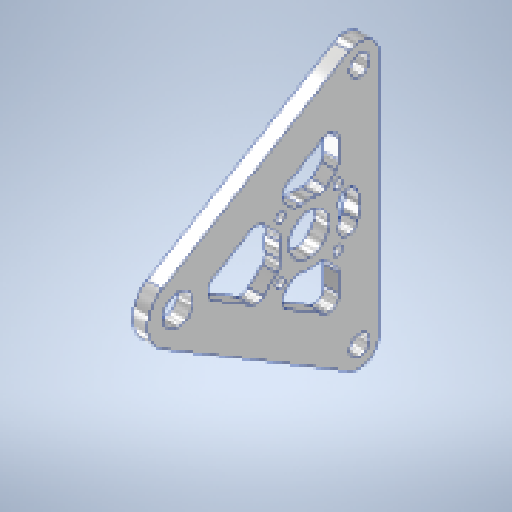
# Autodesk Inventor part: Frame (Motor Side)
Saved by Autodesk Inventor 2023.2 (Build 272271000, 271)
## iProperties
Created: 2022-05-22
Part Number: Frame (Motor Side)
Material: Aluminum 6061
Document SubType Name: Modeling
Designer: Nathan Cai
Density: 2.7 g/cm^3
Appearance: Aluminum - Flat
Mass: 51.1911 g
Surface Area: 97.1122 cm^2
Volume: 18.9597 cm^3
Author: Nathan Cai
Autodesk Inventor part; units mm, degrees
ref_plane "YZ Plane" through (0, 0, 0) normal (1, 0, 0) x (0, 1, 0)
ref_plane "XZ Plane" through (0, 0, 0) normal (0, 1, 0) x (-1, 0, 0)
ref_plane "XY Plane" through (0, 0, 0) normal (0, 0, 1) x (1, 0, 0)
sketch "Sketch1" plane through (0, 0, 0) normal (1, 0, 0) x (0, 1, 0)
  circle A0 centre (0, 0) radius 6.35
  circle A1 centre (0, 0) radius 22.225
  line L0 (0, 0) -> (0, 41.275) construction
  circle A2 centre (0, 41.275) radius 4.7625
  circle A3 centre (0, 41.275) radius 76.2 construction
  circle A4 centre (0, 41.275) radius 9.525
  line L1 (0, -15.875) -> (38.1, -15.875) construction
  circle A5 centre (38.1, -15.875) radius 3.175
  arc A6 (32.6593, -19.1494) -> (43.5407, -12.6006) centre (38.1, -15.875) ccw
  line L2 (8.161, 46.1865) -> (43.5407, -12.6006)
  line L3 (1.9103, 31.9435) -> (32.6593, -19.1494)
  circle A7 centre (-38.1, -15.875) radius 3.175
  arc A8 (-43.5407, -12.6006) -> (-32.6593, -19.1494) centre (-38.1, -15.875) ccw
  line L4 (-8.161, 46.1865) -> (-43.5407, -12.6006)
  line L5 (-1.9103, 31.9435) -> (-32.6593, -19.1494)
  line L6 (0, 0) -> (9.5, 0) construction
  line L7 (0, 0) -> (12.7, 0) construction
  line L8 (0, 0) -> (4.3437, -11.9341)
  line L9 (38.1, -15.875) -> (7.351, 35.2179) construction
  line L10 (-9, 9) -> (9, 9) construction
  arc A9 (3.287, 12.2673) -> (-3.287, 12.2673) centre (0, 0) ccw construction
  arc A10 (4.1088, 15.3341) -> (-4.1088, 15.3341) centre (0, 0) ccw
  arc A11 (2.4653, 9.2004) -> (-2.4653, 9.2004) centre (0, 0) ccw
  arc A12 (2.4653, 9.2004) -> (4.1088, 15.3341) centre (3.287, 12.2673) ccw
  arc A13 (-4.1088, 15.3341) -> (-2.4653, 9.2004) centre (-3.287, 12.2673) ccw
  line L11 (0, 0) -> (-3.287, 12.2673) construction
  line L12 (0, 0) -> (3.287, 12.2673) construction
  arc A14 (-9.2004, 2.4653) -> (-9.2004, -2.4653) centre (0, 0) ccw
  arc A15 (-9.2004, 2.4653) -> (-15.3341, 4.1088) centre (-12.2673, 3.287) ccw
  arc A16 (-15.3341, -4.1088) -> (-9.2004, -2.4653) centre (-12.2673, -3.287) ccw
  arc A17 (-12.2673, 3.287) -> (-12.2673, -3.287) centre (0, 0) ccw construction
  arc A18 (-15.3341, 4.1088) -> (-15.3341, -4.1088) centre (0, 0) ccw
  arc A19 (-2.4653, -9.2004) -> (2.4653, -9.2004) centre (0, 0) ccw
  arc A20 (-2.4653, -9.2004) -> (-4.1088, -15.3341) centre (-3.287, -12.2673) ccw
  arc A21 (4.1088, -15.3341) -> (2.4653, -9.2004) centre (3.287, -12.2673) ccw
  arc A22 (-3.287, -12.2673) -> (3.287, -12.2673) centre (0, 0) ccw construction
  arc A23 (-4.1088, -15.3341) -> (4.1088, -15.3341) centre (0, 0) ccw
  arc A24 (9.2004, -2.4653) -> (9.2004, 2.4653) centre (0, 0) ccw
  arc A25 (9.2004, -2.4653) -> (15.3341, -4.1088) centre (12.2673, -3.287) ccw
  arc A26 (15.3341, 4.1088) -> (9.2004, 2.4653) centre (12.2673, 3.287) ccw
  arc A27 (12.2673, -3.287) -> (12.2673, 3.287) centre (0, 0) ccw construction
  arc A28 (15.3341, -4.1088) -> (15.3341, 4.1088) centre (0, 0) ccw
  line L13 (38.1, -22.225) -> (-38.1, -22.225)
  line L14 (26.8671, -9.525) -> (-26.8671, -9.525)
  line L15 (-11.5072, 15.9973) -> (-5.5321, 10.0222)
  line L16 (11.5072, 15.9973) -> (5.5321, 10.0222)
  line L17 (14.8811, 10.391) -> (10.0222, 5.5321)
  line L18 (-14.8811, 10.391) -> (-10.0222, 5.5321)
  line L19 (-10.0222, -5.5321) -> (-14.0151, -9.525)
  line L20 (10.0222, -5.5321) -> (14.0151, -9.525)
  circle A29 centre (0, 0) radius 8 construction
  line L21 (0, 0) -> (-5.6569, 5.6569) construction
  circle A30 centre (-5.6569, 5.6569) radius 1.5
  circle A31 centre (0, 0) radius 9.5 construction
  circle A32 centre (6.7175, 6.7175) radius 1.5
  line L22 (6.7175, 6.7175) -> (0, 0) construction
  circle A33 centre (0, 0) radius 12.5 construction
  circle A34 centre (-8.8388, 8.8388) radius 1.5
  circle A35 centre (5.6569, -5.6569) radius 1.5
  circle A36 centre (8.8388, -8.8388) radius 1.5
  circle A37 centre (-6.7175, -6.7175) radius 1.5
  point P0 (9.2604, -20.2038)
  point P1 (-8.161, 46.1865)
  point P2 (-1.9103, 31.9435)
  point P3 (-8.5688, -20.5067)
  point P4 (-20.0805, -9.525)
  point P5 (20.0805, -9.525)
  point P6 (0, -22.225)
  point P7 (5.5321, 10.0222)
  point P8 (-14.8811, 10.391)
  point P9 (-10.0222, 5.5321)
  point P10 (-13.1031, -6.35)
  point P11 (13.1031, -6.35)
  point P12 (12.0702, 18.6618)
  point P13 (0, 22.225)
  point P14 (-12.0702, 18.6618)
  point P15 (8.8708, 20.3779)
  point P16 (22.1597, -1.703)
  point P17 (-22.1597, -1.703)
  point P18 (-8.8708, 20.3779)
  point P19 (14.0151, -9.525)
  point P20 (10.0222, -5.5321)
  dimension "d1" = 44.45
  dimension "d65" = 16
  dimension "d68" = 19
  dimension "d70" = 25
  dimension "d0" = 12.7
  dimension "d3" = 9.525
  dimension "d4" = 152.4
  dimension "d5" = 19.05
  dimension "d6" = 38.1
  dimension "d7" = 6.35
  dimension "d8" = 12.7
  dimension "d10" = 12.7
  dimension "d35" = 70
  dimension "d46" = 12.7
  dimension "d47" = 30
  dimension "d48" = 6.35
  dimension "d52" = 360
  dimension "d58" = 15.875
  dimension "d59" = 57.15
  dimension "d63" = 45
  dimension "d66" = 45
  dimension "d67" = 3
  dimension "d69" = 3
  dimension "d71" = 3
  dimension "d74" = 360
  constraints: 52 point on circle, 46 end point, 34 centre point, 16 coincident, 13 tangent, 12 symmetric about line, 8 point on line, 4 horizontal, 3 parallel, 2 perpendicular, 1 vertical, 80 other
  measures "d0" diameter of A0
  measures "d3" diameter of A2
  measures "d4" diameter of A3
  measures "d5" diameter of A4
  measures "d6" distance of L1.start L1.end
  measures "d7" diameter of A5
  measures "d8" diameter of A6
  measures "d10" distance between parallel lines of L2 L3
  measures "d35" angle of L6 L8
  measures "d46" radius of A9
  measures "d47" angle of L12 L11
  measures "d48" diameter of A13
  measures "d58" distance from line of point (0, 0) L1
  measures "d59" distance from line of A2.centre L1
  measures "d63" angle of L14 L19
  measures "d66" angle of L0 L21
  measures "d67" diameter of A30
  measures "d69" diameter of A32
  measures "d71" diameter of A34
extrude "Extrusion1" add sketch "Sketch1" along normal blind 4.7625 contours A1 L3 | A1 L3 A4 L2 A6 | L5 A1 | A1 L5 A8 L4 A4 | A4 | L3 L17 A26 A24 A25 L20 L14 A36 A21 A19 A20 L19 A16 A14 A15 L18 L5 L15 A13 A11 A12 L16 | L14 L3 A6 L13 A1 | A1 L14 A20 A23 A21 A36 | L13 A8 L5 L14 A1 | L14 A21 A23 A20 | A20 A19 L14 | L14 L8 A21 | A19 A21 L8 L14
fillet "Fillet2" radius 3.175 10 edges at (2.3813, 1.9103, 31.9435) (2.3813, -1.9103, 31.9435) (2.3813, 14.8811, 10.391) (2.3813, 11.5072, 15.9973) (2.3813, 26.8671, -9.525) (2.3813, 14.0151, -9.525) (2.3813, -14.0151, -9.525) (2.3813, -26.8671, -9.525) (2.3813, -14.8811, 10.391) (2.3813, -11.5072, 15.9973)
equation "\"d10\" = d8"
body "Solid1"
